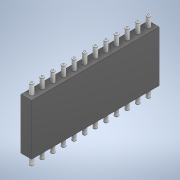
# Autodesk Inventor part: Feather 16-Pin Header
Saved by Autodesk Inventor 2021 (Build 250183000, 183)
## iProperties
Created: 2022-02-21
Part Number: Feather 16-Pin Header
Material: Generic
Document SubType Name: Modeling
Designer: maxsm
Density: 1 g/cm^3
Appearance: Default
Author: maxsm
Autodesk Inventor part; units mm, degrees
ref_plane "YZ Plane" through (0, 0, 0) normal (1, 0, 0) x (0, 1, 0)
ref_plane "XZ Plane" through (0, 0, 0) normal (0, 1, 0) x (-1, 0, 0)
ref_plane "XY Plane" through (0, 0, 0) normal (0, 0, 1) x (1, 0, 0)
sketch "Sketch1" plane through (0, 0, 0) normal (0, 1, 0) x (-1, 0, 0)
  line L0 (0, 0) -> (-2.54, 0)
  line L1 (-2.54, 0) -> (-2.54, -30.48)
  line L2 (-2.54, -30.48) -> (0, -30.48)
  line L3 (0, -30.48) -> (0, 0)
  dimension "d0" = 30.48
  dimension "d1" = 2.54
  constraints: 8 end point, 2 parallel, 1 horizontal, 1 perpendicular
  measures "d0" distance between parallel lines of L2 L0
  measures "d1" distance between parallel lines of L3 L1
extrude "Extrusion1" add sketch "Sketch1" along normal blind 12.192
sketch "Sketch2" plane through (0, 12.192, 0) normal (0, 1, 0) x (1, 0, 0)
  circle A0 centre (1.27, 1.27) radius 0.45
  line L0 (0, 0) -> (2.54, 0) projected
  line L1 (0, 30.48) -> (0, 0) projected
  dimension "d4" = 0.9
  dimension "d5" = 1.27
  dimension "d6" = 1.27
  constraints: 1 centre point
  measures "d4" diameter of A0
  measures "d5" distance from line of L0 A0.centre
  measures "d6" distance from line of A0.centre L1
extrude "Extrusion2" add sketch "Sketch2" along normal blind 2.54
fillet "Fillet1" radius 0.254 1 edges at (0.82, 14.732, -1.27)
pattern_linear "Rectangular Pattern1" count 12 spacing 2.54 along (0, 0, -1) of "Extrusion2", "Fillet1"
ref_plane "Work Plane1" through (0, 6.096, 0) normal (0, 1, 0) x (1, 0, 0)
mirror "Mirror1" about plane through (0, 6.096, 0) normal (0, 1, 0) of "Extrusion2", "Fillet1", "Rectangular Pattern1"
body "Solid1"
